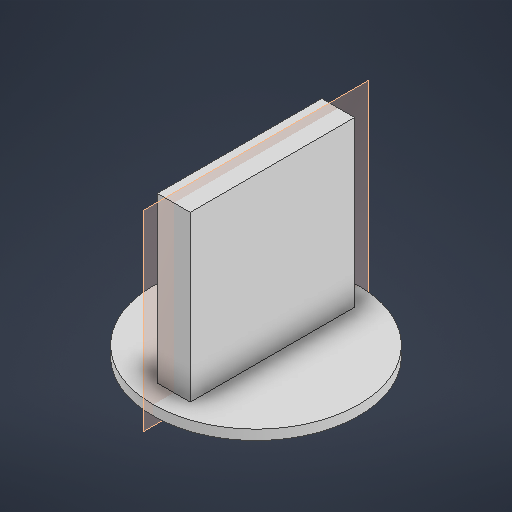
# Autodesk Inventor part: TestBushButton
Saved by Autodesk Inventor 2026 (Build 300175000, 175)
## iProperties
Created: 2025-05-22
Part Number: TestBushButton
Material: Generic
Document SubType Name: Modeling
Designer: Riley
Density: 1 g/cm^3
Appearance: Default
Author: Riley
Autodesk Inventor part; units mm, degrees
ref_plane "XZ Plane" through (0, 0, 0) normal (0, 1, 0) x (-1, 0, 0)
ref_plane "XY Plane" through (0, 0, 0) normal (0, 0, 1) x (1, 0, 0)
sketch "Sketch1" plane through (0, 0, 0) normal (0, 1, 0) x (-1, 0, 0)
  circle A0 centre (0, 0) radius 12.5
  dimension "d0" = 25
  constraints: 1 centre point, 1 coincident
  measures "d0" diameter of A0
extrude "Extrusion1" add sketch "Sketch1" along normal blind 1.2
sketch "Sketch3" plane through (0, 0, 0) normal (1, 0, 0) x (0, 1, 0)
  line L0 (1.2, -12.5) -> (1.2, 12.5) projected
  line L1 (0, -12.5) -> (0, 12.5) projected
  line L2 (1.2, 10) -> (21.2, 10)
  line L3 (21.2, 10) -> (21.2, -10)
  line L4 (21.2, -10) -> (1.2, -10)
  line L5 (1.2, -10) -> (1.2, 10)
  circle A0 centre (11.2, 0) radius 7.5
  point P0 (0, 0)
  point P1 (1.2, -10)
  point P2 (1.2, -10)
  dimension "d3" = 20
  dimension "d4" = 20
  dimension "d5" = 2.5
  dimension "d6" = 15
  constraints: 8 end point, 2 parallel, 1 centre point, 1 horizontal, 1 perpendicular, 1 point on line
  measures "d3" distance of L3.end L4.end
  measures "d4" distance of L2.end L3.end
  measures "d5" distance from line of L0.end L2
  measures "d6" diameter of A0
extrude "Extrusion2" add sketch "Sketch3" along normal mid plane 4
sketch "Sketch4" plane through (2, 0, 0) normal (1, 0, 0) x (0, 0, -1)
  line L0 (-10, 21.2) -> (-10, 1.2) projected
  line L1 (10, 1.2) -> (-10, 1.2) projected
  line L2 (10, 1.2) -> (10, 21.2) projected
  line L3 (10, 21.2) -> (-10, 21.2) projected
  circle A0 centre (0, 11.2) radius 7.5 projected
  circle A1 centre (0, 11.2) radius 7.5
  point P0 (0, 0)
  constraints: 1 centre point, 1 coincident, 1 concentric
extrude "Extrusion3" add sketch "Sketch4" against normal blind 0.4 contours A0
sketch "Sketch5" plane through (1.6, 11.2, 0) normal (-1, 0, 0) x (0, 0, 1)
  line L0 (10, -10) -> (10, 10) projected
  line L1 (10, 10) -> (-10, 10) projected
  line L2 (-10, 10) -> (-10, -10) projected
  line L3 (10, -10) -> (-10, -10) projected
  circle A0 centre (0, 0) radius 7.5 projected
  circle A1 centre (0, 0) radius 2.5
  point P0 (0, -11.2)
  point P1 (0.000179, -7.5)
  dimension "d17" = 5
  constraints: 1 centre point, 2 other
  measures "d17" diameter of A1
extrude "Extrusion4" add sketch "Sketch5" along normal up to surface (3.6 mm away) contours A1
sketch "Sketch7" plane through (-2, 11.2, 0) normal (-1, 0, 0) x (0, 0, 1)
  circle A0 centre (0, 0) radius 7.5
  line L0 (-0.006904, -7.499997) -> (2.356254, -0.835503)
  line L1 (-0.006904, -7.499997) -> (-2.357789, -0.831163)
  circle A1 centre (0, 0) radius 2.5
  circle A2 centre (0, 0) radius 2.5
  point P0 (0, -11.2)
  point P1 (2.356254, -0.835503)
  point P2 (-2.357789, -0.831163)
  constraints: 4 end point, 2 point on circle, 2 tangent, 2 other
sketch "Sketch7 outline for Extrusion5" plane through (-2, 11.2, 0) normal (-1, 0, 0) x (0, 0, 1)
  arc A0 (2.356254, -0.835503) -> (-2.357789, -0.831163) centre (0, 0) cw
  line L0 (-0.006904, -7.499997) -> (2.356254, -0.835503)
  line L1 (-2.357789, -0.831163) -> (-0.006904, -7.499997)
extrude "Extrusion5" add sketch "Sketch7 outline for Extrusion5" against normal blind 0.8
body "Solid1"
